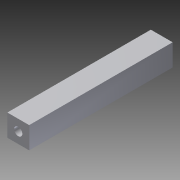
# Autodesk Inventor part: Spacer
Saved by Autodesk Inventor 2015 (Build 190159000, 159)
## iProperties
Created: 2016-03-09
Part Number: Spacer
Material: ABS Plastic
Document SubType Name: Modeling
Designer: 709252
Density: 1.06 g/cm^3
Appearance: Smooth - White
Mass: 2.12716 g
Surface Area: 17.533 cm^2
Volume: 2.00676 cm^3
Author: 709252
Autodesk Inventor part; units mm, degrees
ref_plane "YZ Plane" through (0, 0, 0) normal (1, 0, 0) x (0, 1, 0)
ref_plane "XZ Plane" through (0, 0, 0) normal (0, 1, 0) x (-1, 0, 0)
ref_plane "XY Plane" through (0, 0, 0) normal (0, 0, 1) x (1, 0, 0)
sketch "Sketch1" plane through (0, 0, 0) normal (0, 1, 0) x (-1, 0, 0)
  line L0 (0, 0) -> (-7, 0)
  line L1 (-7, 0) -> (-7, -7)
  line L2 (-7, -7) -> (0, -7)
  line L3 (0, -7) -> (0, 0)
  dimension "d0" = 7
  dimension "d1" = 7
  constraints: 8 end point, 2 parallel, 1 horizontal, 1 perpendicular
  measures "d0" distance of L2.end L1.end
  measures "d1" distance of L1.end L0.end
extrude "Extrusion1" add sketch "Sketch1" along normal blind 46
sketch "Sketch2" plane through (0, 46, 0) normal (0, 1, 0) x (1, 0, 0)
  line L0 (0, 7) -> (0, 0) projected
  line L1 (0, 3.5) -> (7, 3.5)
  line L2 (7, 0) -> (7, 7) projected
  line L3 (7, 7) -> (0, 7) projected
  line L4 (3.5, 7) -> (3.5, 0)
  line L5 (0, 0) -> (7, 0) projected
  point P0 (3.5, 3.5)
  constraints: 5 midpoint, 4 end point
hole "Hole1" at (3.5, 46, -3.5) direction (0, -1, 0) diameter 2.616 end through all
body "Solid1"
